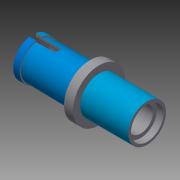
# Autodesk Inventor part: Axle finsihed
Saved by Autodesk Inventor 2015 (Build 190159000, 159)
## iProperties
Created: 2014-10-06
Part Number: Axle finsihed
Material: Generic
Document SubType Name: Modeling
Designer: mbmentzer
Density: 1 g/cm^3
Appearance: Default
Author: mbmentzer
Autodesk Inventor part; units mm, degrees
ref_plane "YZ Plane" through (0, 0, 0) normal (1, 0, 0) x (0, 1, 0)
ref_plane "XZ Plane" through (0, 0, 0) normal (0, 1, 0) x (-1, 0, 0)
ref_plane "XY Plane" through (0, 0, 0) normal (0, 0, 1) x (1, 0, 0)
sketch "Sketch1" plane through (0, 0, 0) normal (0, 0, 1) x (1, 0, 0)
  line L0 (0, 3.81) -> (0, 3.1858)
  line L1 (21.082, 2.413) -> (12.7, 2.413)
  line L2 (12.7, 2.413) -> (12.7, 0)
  line L3 (21.082, 2.413) -> (21.082, 3.175)
  line L4 (21.082, 3.175) -> (22.352, 3.175)
  line L5 (22.352, 3.683) -> (12.954, 3.683)
  line L6 (12.954, 3.683) -> (12.954, 5.08)
  line L7 (22.352, 3.175) -> (22.352, 3.683)
  line L8 (11.176, 0) -> (12.7, 0)
  line L9 (6.35, 2.413) -> (11.176, 2.413)
  line L10 (11.176, 2.413) -> (11.176, 0)
  line L11 (0, 3.81) -> (1.27, 3.81)
  line L12 (1.27, 3.81) -> (1.27, 3.556)
  line L13 (1.27, 3.556) -> (11.176, 3.683)
  line L14 (12.954, 5.08) -> (11.176, 5.08)
  line L15 (11.176, 5.08) -> (11.176, 3.683)
  line L16 (6.35, 2.413) -> (6.35, 3.1858)
  line L17 (6.35, 3.1858) -> (0, 3.1858)
  point P0 (0, 0)
  dimension "d3" = 1.27
  dimension "d8" = 1.778
  dimension "d9" = 1.27
  dimension "d11" = 4.826
  dimension "d12" = 8.382
  dimension "d13" = 22.352
  dimension "d14" = 6.35
  dimension "d15" = 3.683
  dimension "d16" = 2.413
  dimension "d17" = 3.175
  dimension "d18" = 3.683
  dimension "d19" = 3.81
  dimension "d20" = 0.254
  dimension "d21" = 3.1858
  dimension "d22" = 2.413
  dimension "d23" = 5.08
  dimension "d24" = 11.176
  dimension "d25" = 2.413
  constraints: 36 end point, 7 horizontal, 5 vertical, 4 perpendicular, 1 other
  measures "d3" distance of L3.end L4.end
  measures "d8" distance of L6.end L14.end
  measures "d9" distance of L0.start L11.end
  measures "d11" distance of L9.start L9.end
  measures "d12" horizontal distance of L1.start L2.end
  measures "d13" distance between parallel lines of L7 L0
  measures "d14" horizontal distance of L0.end L9.start
  measures "d15" distance of L13.end L8.start
  measures "d16" vertical distance of L1.start L2.end
  measures "d17" vertical distance of L2.end L4.end
  measures "d18" vertical distance of L2.end L5.start
  measures "d19" vertical distance of L0.start L8.start
  measures "d20" distance of L11.end L12.end
  measures "d21" vertical distance of L8.start L0.end
  measures "d22" vertical distance of L8.start L9.start
  measures "d23" distance of L8.start L14.end
  measures "d24" horizontal distance of L14.end L0.start
  measures "d25" distance of L1.end L2.end
revolve "Revolution1" add sketch "Sketch1" angle 360 about axis through (11.176, 0, 0) along (1, 0, 0)
sketch "Sketch2" plane through (0, 0, 0) normal (-1, 0, 0) x (0, 0, 1)
  line L0 (-0.6046, -5.7758) -> (0.6365, -5.7758)
  line L1 (0.6365, -5.7758) -> (0.6365, 5.9031)
  line L2 (0.6365, 5.9031) -> (-0.6046, 5.9031)
  line L3 (-0.6046, 5.9031) -> (-0.6046, -5.7758)
  point P0 (0, 0)
  constraints: 8 end point, 2 parallel, 1 horizontal, 1 perpendicular
extrude "Extrusion1" cut sketch "Sketch2" against normal blind 5
body "Solid1"
